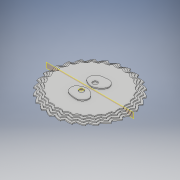
# Autodesk Inventor part: susuwatari
Saved by Autodesk Inventor 2018 (Build 220112000, 112)
## iProperties
Created: 2017-10-30
Part Number: susuwatari
Material: Generic
Document SubType Name: Modeling
Designer: lewisw19
Density: 1 g/cm^3
Appearance: Default
Author: lewisw19
Autodesk Inventor part; units mm, degrees
ref_plane "YZ Plane" through (0, 0, 0) normal (1, 0, 0) x (0, 1, 0)
ref_plane "XZ Plane" through (0, 0, 0) normal (0, 1, 0) x (-1, 0, 0)
sketch "Sketch1" plane through (0, 0, 0) normal (0, 1, 0) x (-1, 0, 0)
  arc A0 (255.3081, 0.1624) -> (269.4241, 48.2355) centre (181.7679, 47.8654) ccw
  arc A1 (248.6593, 60.0433) -> (269.4241, 48.2355) centre (269.4545, 72.4509) ccw
  arc A2 (248.6593, 60.0433) -> (250.9174, 108.9566) centre (165.7093, 88.3816) ccw
  arc A3 (228.0167, 115.6292) -> (250.9174, 108.9566) centre (245.3625, 132.5263) ccw
  arc A4 (228.0167, 115.6292) -> (218.9338, 163.7448) centre (140.7674, 124.074) ccw
  arc A5 (195.1456, 164.9347) -> (218.9338, 163.7448) centre (208.0931, 185.3981) ccw
  arc A6 (195.1456, 164.9347) -> (175.2114, 209.6586) centre (108.3007, 153.0308) ccw
  arc A7 (151.829, 205.3171) -> (175.2114, 209.6586) centre (159.6693, 228.2283) ccw
  arc A8 (151.829, 205.3171) -> (122.1181, 244.2383) centre (70.0702, 173.7063) ccw
  arc A9 (100.4094, 234.6175) -> (122.1181, 244.2383) centre (102.7124, 258.7232) ccw
  arc A10 (100.4094, 234.6175) -> (62.5234, 265.6378) centre (28.1443, 185.0038) ccw
  arc A11 (43.6616, 251.2759) -> (62.5234, 265.6378) centre (40.3004, 275.2569) ccw
  arc A12 (43.6616, 251.2759) -> (-0.3569, 272.7229) centre (-15.2139, 186.3341) ccw
  arc A13 (-15.3568, 254.4145) -> (-0.3569, 272.7229) centre (-24.1992, 276.9578) ccw
  arc A14 (-15.3568, 254.4145) -> (-63.1348, 265.132) centre (-57.6686, 177.6456) ccw
  arc A15 (-73.4706, 243.884) -> (-63.1348, 265.132) centre (-87.311, 263.7543) ccw
  arc A16 (-73.4706, 243.884) -> (-122.4324, 243.2943) centre (-96.9378, 159.4266) ccw
  arc A17 (-127.5582, 220.2704) -> (-122.4324, 243.2943) centre (-145.6392, 236.3783) ccw
  arc A18 (-127.5582, 220.2704) -> (-175.0642, 208.4052) centre (-130.9156, 132.6777) ccw
  arc A19 (-174.7194, 184.8623) -> (-175.0642, 208.4052) centre (-196.0506, 196.3238) ccw
  arc A20 (-174.7194, 184.8623) -> (-218.2085, 162.3613) centre (-157.786, 98.8564) ccw
  arc A21 (-212.4309, 139.5804) -> (-218.2085, 162.3613) centre (-235.8431, 145.7657) ccw
  arc A22 (-212.4309, 139.5804) -> (-249.5587, 107.6566) centre (-176.1197, 59.7979) ccw
  arc A23 (-238.6819, 86.8731) -> (-249.5587, 107.6566) centre (-262.8907, 87.4416) ccw
  arc A24 (-238.6819, 86.8731) -> (-267.4468, 47.2476) centre (-184.9504, 17.6151) ccw
  arc A25 (-252.0702, 29.5327) -> (-267.4468, 47.2476) centre (-275.7576, 24.5029) ccw
  arc A26 (-252.0702, 29.5327) -> (-267.6415, 0.1624) centre (-183.815, -25.4671) ccw
  arc A27 (269.4241, -47.9107) -> (255.3081, 0.1624) centre (181.7679, -47.5406) ccw
  arc A28 (269.4241, -47.9107) -> (248.6593, -59.7185) centre (269.4545, -72.1261) ccw
  arc A29 (250.9174, -108.6318) -> (248.6593, -59.7185) centre (165.7093, -88.0568) ccw
  arc A30 (250.9174, -108.6318) -> (228.0167, -115.3044) centre (245.3625, -132.2015) ccw
  arc A31 (218.9338, -163.42) -> (228.0167, -115.3044) centre (140.7674, -123.7492) ccw
  arc A32 (218.9338, -163.42) -> (195.1456, -164.6099) centre (208.0931, -185.0733) ccw
  arc A33 (175.2114, -209.3338) -> (195.1456, -164.6099) centre (108.3007, -152.706) ccw
  arc A34 (175.2114, -209.3338) -> (151.829, -204.9923) centre (159.6693, -227.9035) ccw
  arc A35 (122.1181, -243.9135) -> (151.829, -204.9923) centre (70.0702, -173.3815) ccw
  arc A36 (122.1181, -243.9135) -> (100.4094, -234.2927) centre (102.7124, -258.3984) ccw
  arc A37 (62.5234, -265.313) -> (100.4094, -234.2927) centre (28.1443, -184.679) ccw
  arc A38 (62.5234, -265.313) -> (43.6616, -250.9511) centre (40.3004, -274.9321) ccw
  arc A39 (-0.3569, -272.3981) -> (43.6616, -250.9511) centre (-15.2139, -186.0093) ccw
  arc A40 (-0.3569, -272.3981) -> (-15.3568, -254.0897) centre (-24.1992, -276.633) ccw
  arc A41 (-63.1348, -264.8072) -> (-15.3568, -254.0897) centre (-57.6686, -177.3208) ccw
  arc A42 (-63.1348, -264.8072) -> (-73.4706, -243.5592) centre (-87.311, -263.4295) ccw
  arc A43 (-122.4324, -242.9695) -> (-73.4706, -243.5592) centre (-96.9378, -159.1018) ccw
  arc A44 (-122.4324, -242.9695) -> (-127.5582, -219.9456) centre (-145.6392, -236.0535) ccw
  arc A45 (-175.0642, -208.0804) -> (-127.5582, -219.9456) centre (-130.9156, -132.3529) ccw
  arc A46 (-175.0642, -208.0804) -> (-174.7194, -184.5375) centre (-196.0506, -195.999) ccw
  arc A47 (-218.2085, -162.0365) -> (-174.7194, -184.5375) centre (-157.786, -98.5316) ccw
  arc A48 (-218.2085, -162.0365) -> (-212.4309, -139.2556) centre (-235.8431, -145.4409) ccw
  arc A49 (-249.5587, -107.3318) -> (-212.4309, -139.2556) centre (-176.1197, -59.4731) ccw
  arc A50 (-249.5587, -107.3318) -> (-238.6819, -86.5483) centre (-262.8907, -87.1168) ccw
  arc A51 (-267.4468, -46.9228) -> (-238.6819, -86.5483) centre (-184.9504, -17.2903) ccw
  arc A52 (-267.4468, -46.9228) -> (-252.0702, -29.2079) centre (-275.7576, -24.1781) ccw
  arc A53 (-267.6415, 0.1624) -> (-252.0702, -29.2079) centre (-183.815, 25.7919) ccw
  point P0 (0, 0)
  constraints: 108 point on circle, 54 centre point
extrude "Extrusion1" add sketch "Sketch1" along normal blind 6.35
sketch "Sketch2" plane through (0, 6.35, 0) normal (0, 1, 0) x (1, 0, 0)
  arc A0 (-255.3081, -0.1624) -> (-269.4241, -48.2355) centre (-181.7679, -47.8654) ccw projected
  arc A1 (-248.6593, -60.0433) -> (-269.4241, -48.2355) centre (-269.4545, -72.4509) ccw projected
  arc A2 (-248.6593, -60.0433) -> (-250.9174, -108.9566) centre (-165.7093, -88.3816) ccw projected
  arc A3 (-228.0167, -115.6292) -> (-250.9174, -108.9566) centre (-245.3625, -132.5263) ccw projected
  arc A4 (-228.0167, -115.6292) -> (-218.9338, -163.7448) centre (-140.7674, -124.074) ccw projected
  arc A5 (-195.1456, -164.9347) -> (-218.9338, -163.7448) centre (-208.0931, -185.3981) ccw projected
  arc A6 (-195.1456, -164.9347) -> (-175.2114, -209.6586) centre (-108.3007, -153.0308) ccw projected
  arc A7 (-151.829, -205.3171) -> (-175.2114, -209.6586) centre (-159.6693, -228.2283) ccw projected
  arc A8 (-151.829, -205.3171) -> (-122.1181, -244.2383) centre (-70.0702, -173.7063) ccw projected
  arc A9 (-100.4094, -234.6175) -> (-122.1181, -244.2383) centre (-102.7124, -258.7232) ccw projected
  arc A10 (-100.4094, -234.6175) -> (-62.5234, -265.6378) centre (-28.1443, -185.0038) ccw projected
  arc A11 (-43.6616, -251.2759) -> (-62.5234, -265.6378) centre (-40.3004, -275.2569) ccw projected
  arc A12 (-43.6616, -251.2759) -> (0.3569, -272.7229) centre (15.2139, -186.3341) ccw projected
  arc A13 (15.3568, -254.4145) -> (0.3569, -272.7229) centre (24.1992, -276.9578) ccw projected
  arc A14 (15.3568, -254.4145) -> (63.1348, -265.132) centre (57.6686, -177.6456) ccw projected
  arc A15 (73.4706, -243.884) -> (63.1348, -265.132) centre (87.311, -263.7543) ccw projected
  arc A16 (73.4706, -243.884) -> (122.4324, -243.2943) centre (96.9378, -159.4266) ccw projected
  arc A17 (127.5582, -220.2704) -> (122.4324, -243.2943) centre (145.6392, -236.3783) ccw projected
  arc A18 (127.5582, -220.2704) -> (175.0642, -208.4052) centre (130.9156, -132.6777) ccw projected
  arc A19 (174.7194, -184.8623) -> (175.0642, -208.4052) centre (196.0506, -196.3238) ccw projected
  arc A20 (174.7194, -184.8623) -> (218.2085, -162.3613) centre (157.786, -98.8564) ccw projected
  arc A21 (212.4309, -139.5804) -> (218.2085, -162.3613) centre (235.8431, -145.7657) ccw projected
  arc A22 (212.4309, -139.5804) -> (249.5587, -107.6566) centre (176.1197, -59.7979) ccw projected
  arc A23 (238.6819, -86.8731) -> (249.5587, -107.6566) centre (262.8907, -87.4416) ccw projected
  arc A24 (238.6819, -86.8731) -> (267.4468, -47.2476) centre (184.9504, -17.6151) ccw projected
  arc A25 (252.0702, -29.5327) -> (267.4468, -47.2476) centre (275.7576, -24.5029) ccw projected
  arc A26 (252.0702, -29.5327) -> (267.6415, -0.1624) centre (183.815, 25.4671) ccw projected
  arc A27 (267.6415, -0.1624) -> (252.0702, 29.2079) centre (183.815, -25.7919) ccw projected
  arc A28 (267.4468, 46.9228) -> (252.0702, 29.2079) centre (275.7576, 24.1781) ccw projected
  arc A29 (267.4468, 46.9228) -> (238.6819, 86.5483) centre (184.9504, 17.2903) ccw projected
  arc A30 (249.5587, 107.3318) -> (238.6819, 86.5483) centre (262.8907, 87.1168) ccw projected
  arc A31 (249.5587, 107.3318) -> (212.4309, 139.2556) centre (176.1197, 59.4731) ccw projected
  arc A32 (218.2085, 162.0365) -> (212.4309, 139.2556) centre (235.8431, 145.4409) ccw projected
  arc A33 (218.2085, 162.0365) -> (174.7194, 184.5375) centre (157.786, 98.5316) ccw projected
  arc A34 (175.0642, 208.0804) -> (174.7194, 184.5375) centre (196.0506, 195.999) ccw projected
  arc A35 (175.0642, 208.0804) -> (127.5582, 219.9456) centre (130.9156, 132.3529) ccw projected
  arc A36 (122.4324, 242.9695) -> (127.5582, 219.9456) centre (145.6392, 236.0535) ccw projected
  arc A37 (122.4324, 242.9695) -> (73.4706, 243.5592) centre (96.9378, 159.1018) ccw projected
  arc A38 (63.1348, 264.8072) -> (73.4706, 243.5592) centre (87.311, 263.4295) ccw projected
  arc A39 (63.1348, 264.8072) -> (15.3568, 254.0897) centre (57.6686, 177.3208) ccw projected
  arc A40 (0.3569, 272.3981) -> (15.3568, 254.0897) centre (24.1992, 276.633) ccw projected
  arc A41 (0.3569, 272.3981) -> (-43.6616, 250.9511) centre (15.2139, 186.0093) ccw projected
  arc A42 (-62.5234, 265.313) -> (-43.6616, 250.9511) centre (-40.3004, 274.9321) ccw projected
  arc A43 (-62.5234, 265.313) -> (-100.4094, 234.2927) centre (-28.1443, 184.679) ccw projected
  arc A44 (-122.1181, 243.9135) -> (-100.4094, 234.2927) centre (-102.7124, 258.3984) ccw projected
  arc A45 (-122.1181, 243.9135) -> (-151.829, 204.9923) centre (-70.0702, 173.3815) ccw projected
  arc A46 (-175.2114, 209.3338) -> (-151.829, 204.9923) centre (-159.6693, 227.9035) ccw projected
  arc A47 (-175.2114, 209.3338) -> (-195.1456, 164.6099) centre (-108.3007, 152.706) ccw projected
  arc A48 (-218.9338, 163.42) -> (-195.1456, 164.6099) centre (-208.0931, 185.0733) ccw projected
  arc A49 (-218.9338, 163.42) -> (-228.0167, 115.3044) centre (-140.7674, 123.7492) ccw projected
  arc A50 (-250.9174, 108.6318) -> (-228.0167, 115.3044) centre (-245.3625, 132.2015) ccw projected
  arc A51 (-250.9174, 108.6318) -> (-248.6593, 59.7185) centre (-165.7093, 88.0568) ccw projected
  arc A52 (-269.4241, 47.9107) -> (-248.6593, 59.7185) centre (-269.4545, 72.1261) ccw projected
  arc A53 (-269.4241, 47.9107) -> (-255.3081, -0.1624) centre (-181.7679, 47.5406) ccw projected
  arc A54 (-234.8822, -59.5084) -> (-240.282, -95.9621) centre (-165.7093, -88.3816) ccw
  arc A55 (-234.8822, -59.5084) -> (-256.0786, -38.044) centre (-269.4545, -72.4509) ccw
  arc A56 (-239.5863, -0.1624) -> (-256.0786, -38.044) centre (-181.7679, -47.8654) ccw
  arc A57 (-256.0786, 37.7192) -> (-239.5863, -0.1624) centre (-181.7679, 47.5406) ccw
  arc A58 (-256.0786, 37.7192) -> (-234.8822, 59.1836) centre (-269.4545, 72.1261) ccw
  arc A59 (-240.282, 95.6373) -> (-234.8822, 59.1836) centre (-165.7093, 88.0568) ccw
  arc A60 (-240.282, 95.6373) -> (-214.7327, 111.5965) centre (-245.3625, 132.2015) ccw
  arc A61 (-211.5818, 148.3231) -> (-214.7327, 111.5965) centre (-140.7674, 123.7492) ccw
  arc A62 (-211.5818, 148.3231) -> (-183.0755, 157.9279) centre (-208.0931, 185.0733) ccw
  arc A63 (-171.5391, 192.9484) -> (-183.0755, 157.9279) centre (-108.3007, 152.706) ccw
  arc A64 (-171.5391, 192.9484) -> (-141.6285, 195.6966) centre (-159.6693, 227.9035) ccw
  arc A65 (-122.3236, 227.1229) -> (-141.6285, 195.6966) centre (-70.0702, 173.3815) ccw
  arc A66 (-122.3236, 227.1229) -> (-92.6332, 222.8856) centre (-102.7124, 258.3984) ccw
  arc A67 (-66.5955, 249.0223) -> (-92.6332, 222.8856) centre (-28.1443, 184.679) ccw
  arc A68 (-66.5955, 249.0223) -> (-38.7336, 238.0499) centre (-40.3004, 274.9321) ccw
  arc A69 (-7.3623, 257.4856) -> (-38.7336, 238.0499) centre (15.2139, 186.0093) ccw
  arc A70 (-7.3623, 257.4856) -> (17.1669, 240.3935) centre (24.1992, 276.633) ccw
  arc A71 (52.1846, 252.0769) -> (17.1669, 240.3935) centre (57.6686, 177.3208) ccw
  arc A72 (52.1846, 252.0769) -> (72.0621, 229.8108) centre (87.311, 263.4295) ccw
  arc A73 (108.8415, 233.1076) -> (72.0621, 229.8108) centre (96.9378, 159.1018) ccw
  arc A74 (108.8415, 233.1076) -> (123.0048, 206.8913) centre (145.6392, 236.0535) ccw
  arc A75 (159.5654, 201.6187) -> (123.0048, 206.8913) centre (130.9156, 132.3529) ccw
  arc A76 (159.5654, 201.6187) -> (167.2656, 172.8868) centre (196.0506, 195.999) ccw
  arc A77 (201.6373, 159.3232) -> (167.2656, 172.8868) centre (157.786, 98.5316) ccw
  arc A78 (201.6373, 159.3232) -> (202.479, 129.6424) centre (235.8431, 145.4409) ccw
  arc A79 (232.8084, 108.5132) -> (202.479, 129.6424) centre (176.1197, 59.4731) ccw
  arc A80 (232.8084, 108.5132) -> (226.7703, 79.4968) centre (262.8907, 87.1168) ccw
  arc A81 (251.4205, 51.9353) -> (226.7703, 79.4968) centre (184.9504, 17.2903) ccw
  arc A82 (251.4205, 51.9353) -> (238.8535, 25.0935) centre (275.7576, 24.1781) ccw
  arc A83 (254.2542, -0.1624) -> (238.8535, 25.0935) centre (183.815, -25.7919) ccw
  arc A84 (238.8535, -25.4183) -> (254.2542, -0.1624) centre (183.815, 25.4671) ccw
  arc A85 (238.8535, -25.4183) -> (251.4205, -52.2601) centre (275.7576, -24.5029) ccw
  arc A86 (226.7703, -79.8216) -> (251.4205, -52.2601) centre (184.9504, -17.6151) ccw
  arc A87 (226.7703, -79.8216) -> (232.8084, -108.838) centre (262.8907, -87.4416) ccw
  arc A88 (202.479, -129.9672) -> (232.8084, -108.838) centre (176.1197, -59.7979) ccw
  arc A89 (202.479, -129.9672) -> (201.6373, -159.648) centre (235.8431, -145.7657) ccw
  arc A90 (167.2656, -173.2116) -> (201.6373, -159.648) centre (157.786, -98.8564) ccw
  arc A91 (167.2656, -173.2116) -> (159.5654, -201.9435) centre (196.0506, -196.3238) ccw
  arc A92 (123.0048, -207.2161) -> (159.5654, -201.9435) centre (130.9156, -132.6777) ccw
  arc A93 (123.0048, -207.2161) -> (108.8415, -233.4324) centre (145.6392, -236.3783) ccw
  arc A94 (72.0621, -230.1356) -> (108.8415, -233.4324) centre (96.9378, -159.4266) ccw
  arc A95 (72.0621, -230.1356) -> (52.1846, -252.4017) centre (87.311, -263.7543) ccw
  arc A96 (17.1669, -240.7183) -> (52.1846, -252.4017) centre (57.6686, -177.6456) ccw
  arc A97 (17.1669, -240.7183) -> (-7.3623, -257.8104) centre (24.1992, -276.9578) ccw
  arc A98 (-38.7336, -238.3747) -> (-7.3623, -257.8104) centre (15.2139, -186.3341) ccw
  arc A99 (-38.7336, -238.3747) -> (-66.5955, -249.3471) centre (-40.3004, -275.2569) ccw
  arc A100 (-92.6332, -223.2104) -> (-66.5955, -249.3471) centre (-28.1443, -185.0038) ccw
  arc A101 (-92.6332, -223.2104) -> (-122.3236, -227.4477) centre (-102.7124, -258.7232) ccw
  arc A102 (-141.6285, -196.0214) -> (-122.3236, -227.4477) centre (-70.0702, -173.7063) ccw
  arc A103 (-141.6285, -196.0214) -> (-171.5391, -193.2732) centre (-159.6693, -228.2283) ccw
  arc A104 (-183.0755, -158.2527) -> (-171.5391, -193.2732) centre (-108.3007, -153.0308) ccw
  arc A105 (-183.0755, -158.2527) -> (-211.5818, -148.6479) centre (-208.0931, -185.3981) ccw
  arc A106 (-214.7327, -111.9213) -> (-211.5818, -148.6479) centre (-140.7674, -124.074) ccw
  arc A107 (-214.7327, -111.9213) -> (-240.282, -95.9621) centre (-245.3625, -132.5263) ccw
  point P0 (0, 0)
  dimension "d10" = 12.7
  constraints: 108 point on circle, 54 centre point, 53 other
  measures "d10" radial gap between concentric circles of A3 A107
extrude "Extrusion2" add sketch "Sketch2" along normal blind 6.35 contours A55 A56 A57 A58 A59 A60 A61 A62 A63 A64 A65 A66 A67 A68 A69 A70 A71 A72 A73 A74 A75 A76 A77 A78 A79 A80 A81 A82 A83 A84 A85 A86 A87 A88 A89 A90 A91 A92 A93 A94 A95 A96 A97 A98 A99 A100 A101 A102 A103 A104 A105 A106 A107 A54
sketch "Sketch3" plane through (0, 12.7, 0) normal (0, 1, 0) x (1, 0, 0)
  arc A0 (-234.8822, -59.5084) -> (-240.282, -95.9621) centre (-165.7093, -88.3816) ccw projected
  arc A1 (-214.7327, -111.9213) -> (-240.282, -95.9621) centre (-245.3625, -132.5263) ccw projected
  arc A2 (-214.7327, -111.9213) -> (-211.5818, -148.6479) centre (-140.7674, -124.074) ccw projected
  arc A3 (-183.0755, -158.2527) -> (-211.5818, -148.6479) centre (-208.0931, -185.3981) ccw projected
  arc A4 (-183.0755, -158.2527) -> (-171.5391, -193.2732) centre (-108.3007, -153.0308) ccw projected
  arc A5 (-141.6285, -196.0214) -> (-171.5391, -193.2732) centre (-159.6693, -228.2283) ccw projected
  arc A6 (-141.6285, -196.0214) -> (-122.3236, -227.4477) centre (-70.0702, -173.7063) ccw projected
  arc A7 (-92.6332, -223.2104) -> (-122.3236, -227.4477) centre (-102.7124, -258.7232) ccw projected
  arc A8 (-92.6332, -223.2104) -> (-66.5955, -249.3471) centre (-28.1443, -185.0038) ccw projected
  arc A9 (-38.7336, -238.3747) -> (-66.5955, -249.3471) centre (-40.3004, -275.2569) ccw projected
  arc A10 (-38.7336, -238.3747) -> (-7.3623, -257.8104) centre (15.2139, -186.3341) ccw projected
  arc A11 (17.1669, -240.7183) -> (-7.3623, -257.8104) centre (24.1992, -276.9578) ccw projected
  arc A12 (17.1669, -240.7183) -> (52.1846, -252.4017) centre (57.6686, -177.6456) ccw projected
  arc A13 (72.0621, -230.1356) -> (52.1846, -252.4017) centre (87.311, -263.7543) ccw projected
  arc A14 (72.0621, -230.1356) -> (108.8415, -233.4324) centre (96.9378, -159.4266) ccw projected
  arc A15 (123.0048, -207.2161) -> (108.8415, -233.4324) centre (145.6392, -236.3783) ccw projected
  arc A16 (123.0048, -207.2161) -> (159.5654, -201.9435) centre (130.9156, -132.6777) ccw projected
  arc A17 (167.2656, -173.2116) -> (159.5654, -201.9435) centre (196.0506, -196.3238) ccw projected
  arc A18 (167.2656, -173.2116) -> (201.6373, -159.648) centre (157.786, -98.8564) ccw projected
  arc A19 (202.479, -129.9672) -> (201.6373, -159.648) centre (235.8431, -145.7657) ccw projected
  arc A20 (202.479, -129.9672) -> (232.8084, -108.838) centre (176.1197, -59.7979) ccw projected
  arc A21 (226.7703, -79.8216) -> (232.8084, -108.838) centre (262.8907, -87.4416) ccw projected
  arc A22 (226.7703, -79.8216) -> (251.4205, -52.2601) centre (184.9504, -17.6151) ccw projected
  arc A23 (238.8535, -25.4183) -> (251.4205, -52.2601) centre (275.7576, -24.5029) ccw projected
  arc A24 (238.8535, -25.4183) -> (254.2542, -0.1624) centre (183.815, 25.4671) ccw projected
  arc A25 (254.2542, -0.1624) -> (238.8535, 25.0935) centre (183.815, -25.7919) ccw projected
  arc A26 (251.4205, 51.9353) -> (238.8535, 25.0935) centre (275.7576, 24.1781) ccw projected
  arc A27 (251.4205, 51.9353) -> (226.7703, 79.4968) centre (184.9504, 17.2903) ccw projected
  arc A28 (232.8084, 108.5132) -> (226.7703, 79.4968) centre (262.8907, 87.1168) ccw projected
  arc A29 (232.8084, 108.5132) -> (202.479, 129.6424) centre (176.1197, 59.4731) ccw projected
  arc A30 (201.6373, 159.3232) -> (202.479, 129.6424) centre (235.8431, 145.4409) ccw projected
  arc A31 (201.6373, 159.3232) -> (167.2656, 172.8868) centre (157.786, 98.5316) ccw projected
  arc A32 (159.5654, 201.6187) -> (167.2656, 172.8868) centre (196.0506, 195.999) ccw projected
  arc A33 (159.5654, 201.6187) -> (123.0048, 206.8913) centre (130.9156, 132.3529) ccw projected
  arc A34 (108.8415, 233.1076) -> (123.0048, 206.8913) centre (145.6392, 236.0535) ccw projected
  arc A35 (108.8415, 233.1076) -> (72.0621, 229.8108) centre (96.9378, 159.1018) ccw projected
  arc A36 (52.1846, 252.0769) -> (72.0621, 229.8108) centre (87.311, 263.4295) ccw projected
  arc A37 (52.1846, 252.0769) -> (17.1669, 240.3935) centre (57.6686, 177.3208) ccw projected
  arc A38 (-7.3623, 257.4856) -> (17.1669, 240.3935) centre (24.1992, 276.633) ccw projected
  arc A39 (-7.3623, 257.4856) -> (-38.7336, 238.0499) centre (15.2139, 186.0093) ccw projected
  arc A40 (-66.5955, 249.0223) -> (-38.7336, 238.0499) centre (-40.3004, 274.9321) ccw projected
  arc A41 (-66.5955, 249.0223) -> (-92.6332, 222.8856) centre (-28.1443, 184.679) ccw projected
  arc A42 (-122.3236, 227.1229) -> (-92.6332, 222.8856) centre (-102.7124, 258.3984) ccw projected
  arc A43 (-122.3236, 227.1229) -> (-141.6285, 195.6966) centre (-70.0702, 173.3815) ccw projected
  arc A44 (-171.5391, 192.9484) -> (-141.6285, 195.6966) centre (-159.6693, 227.9035) ccw projected
  arc A45 (-171.5391, 192.9484) -> (-183.0755, 157.9279) centre (-108.3007, 152.706) ccw projected
  arc A46 (-211.5818, 148.3231) -> (-183.0755, 157.9279) centre (-208.0931, 185.0733) ccw projected
  arc A47 (-211.5818, 148.3231) -> (-214.7327, 111.5965) centre (-140.7674, 123.7492) ccw projected
  arc A48 (-240.282, 95.6373) -> (-214.7327, 111.5965) centre (-245.3625, 132.2015) ccw projected
  arc A49 (-240.282, 95.6373) -> (-234.8822, 59.1836) centre (-165.7093, 88.0568) ccw projected
  arc A50 (-256.0786, 37.7192) -> (-234.8822, 59.1836) centre (-269.4545, 72.1261) ccw projected
  arc A51 (-256.0786, 37.7192) -> (-239.5863, -0.1624) centre (-181.7679, 47.5406) ccw projected
  arc A52 (-239.5863, -0.1624) -> (-256.0786, -38.044) centre (-181.7679, -47.8654) ccw projected
  arc A53 (-234.8822, -59.5084) -> (-256.0786, -38.044) centre (-269.4545, -72.4509) ccw projected
  arc A54 (-119.2108, 211.6063) -> (-130.6715, 187.644) centre (-70.0702, 173.3815) ccw
  arc A55 (-119.2108, 211.6063) -> (-83.8313, 212.516) centre (-102.7124, 258.3984) ccw
  arc A56 (-67.1451, 233.2061) -> (-83.8313, 212.516) centre (-28.1443, 184.679) ccw
  arc A57 (-67.1451, 233.2061) -> (-32.5648, 225.9234) centre (-40.3004, 274.9321) ccw
  arc A58 (-11.5445, 242.2225) -> (-32.5648, 225.9234) centre (15.2139, 186.0093) ccw
  arc A59 (-11.5445, 242.2225) -> (20.3669, 227.1657) centre (24.1992, 276.633) ccw
  arc A60 (44.5952, 238.1897) -> (20.3669, 227.1657) centre (57.6686, 177.3208) ccw
  arc A61 (44.5952, 238.1897) -> (72.118, 216.1975) centre (87.311, 263.4295) ccw
  arc A62 (98.2541, 221.3449) -> (72.118, 216.1975) centre (96.9378, 159.1018) ccw
  arc A63 (98.2541, 221.3449) -> (119.9116, 193.6297) centre (145.6392, 236.0535) ccw
  arc A64 (146.5507, 192.6147) -> (119.9116, 193.6297) centre (130.9156, 132.3529) ccw
  arc A65 (146.5507, 192.6147) -> (161.1886, 160.6955) centre (196.0506, 195.999) ccw
  arc A66 (186.897, 153.5633) -> (161.1886, 160.6955) centre (157.786, 98.5316) ccw
  arc A67 (186.897, 153.5633) -> (193.7454, 119.183) centre (235.8431, 145.4409) ccw
  arc A68 (217.1371, 106.308) -> (193.7454, 119.183) centre (176.1197, 59.4731) ccw
  arc A69 (217.1371, 106.308) -> (215.8514, 71.3372) centre (262.8907, 87.1168) ccw
  arc A70 (235.663, 53.4035) -> (215.8514, 71.3372) centre (184.9504, 17.2903) ccw
  arc A71 (235.663, 53.4035) -> (226.3472, 19.6718) centre (275.7576, 24.1781) ccw
  arc A72 (240.5518, -0.1624) -> (226.3472, 19.6718) centre (183.815, -25.7919) ccw
  arc A73 (226.3472, -19.9966) -> (240.5518, -0.1624) centre (183.815, 25.4671) ccw
  arc A74 (226.3472, -19.9966) -> (235.663, -53.7283) centre (275.7576, -24.5029) ccw
  arc A75 (215.8514, -71.662) -> (235.663, -53.7283) centre (184.9504, -17.6151) ccw
  arc A76 (215.8514, -71.662) -> (217.1371, -106.6328) centre (262.8907, -87.4416) ccw
  arc A77 (193.7454, -119.5077) -> (217.1371, -106.6328) centre (176.1197, -59.7979) ccw
  arc A78 (193.7454, -119.5077) -> (186.897, -153.8881) centre (235.8431, -145.7657) ccw
  arc A79 (161.1886, -161.0203) -> (186.897, -153.8881) centre (157.786, -98.8564) ccw
  arc A80 (161.1886, -161.0203) -> (146.5507, -192.9395) centre (196.0506, -196.3238) ccw
  arc A81 (119.9116, -193.9545) -> (146.5507, -192.9395) centre (130.9156, -132.6777) ccw
  arc A82 (119.9116, -193.9545) -> (98.2541, -221.6697) centre (145.6392, -236.3783) ccw
  arc A83 (72.118, -216.5223) -> (98.2541, -221.6697) centre (96.9378, -159.4266) ccw
  arc A84 (72.118, -216.5223) -> (44.5952, -238.5145) centre (87.311, -263.7543) ccw
  arc A85 (20.3669, -227.4905) -> (44.5952, -238.5145) centre (57.6686, -177.6456) ccw
  arc A86 (20.3669, -227.4905) -> (-11.5445, -242.5473) centre (24.1992, -276.9578) ccw
  arc A87 (-32.5648, -226.2482) -> (-11.5445, -242.5473) centre (15.2139, -186.3341) ccw
  arc A88 (-32.5648, -226.2482) -> (-67.1451, -233.5309) centre (-40.3004, -275.2569) ccw
  arc A89 (-83.8313, -212.8408) -> (-67.1451, -233.5309) centre (-28.1443, -185.0038) ccw
  arc A90 (-83.8313, -212.8408) -> (-119.2108, -211.9311) centre (-102.7124, -258.7232) ccw
  arc A91 (-130.6715, -187.9688) -> (-119.2108, -211.9311) centre (-70.0702, -173.7063) ccw
  arc A92 (-130.6715, -187.9688) -> (-164.9319, -178.8927) centre (-159.6693, -228.2283) ccw
  arc A93 (-170.5576, -152.9515) -> (-164.9319, -178.8927) centre (-108.3007, -153.0308) ccw
  arc A94 (-170.5576, -152.9515) -> (-201.8363, -136.1787) centre (-208.0931, -185.3981) ccw
  arc A95 (-201.3321, -109.6568) -> (-201.8363, -136.1787) centre (-140.7674, -124.074) ccw
  arc A96 (-201.3321, -109.6568) -> (-227.9236, -86.0765) centre (-245.3625, -132.5263) ccw
  arc A97 (-221.3244, -60.4013) -> (-227.9236, -86.0765) centre (-165.7093, -88.3816) ccw
  arc A98 (-221.3244, -60.4013) -> (-241.7736, -31.2749) centre (-269.4545, -72.4509) ccw
  arc A99 (-221.7723, -0.1624) -> (-241.7736, -31.2749) centre (-181.7679, -47.8654) ccw
  arc A100 (-241.7736, 30.9501) -> (-221.7723, -0.1624) centre (-181.7679, 47.5406) ccw
  arc A101 (-241.7736, 30.9501) -> (-221.3244, 60.0765) centre (-269.4545, 72.1261) ccw
  arc A102 (-227.9236, 85.7517) -> (-221.3244, 60.0765) centre (-165.7093, 88.0568) ccw
  arc A103 (-227.9236, 85.7517) -> (-201.3321, 109.332) centre (-245.3625, 132.2015) ccw
  arc A104 (-201.8363, 135.8539) -> (-201.3321, 109.332) centre (-140.7674, 123.7492) ccw
  arc A105 (-201.8363, 135.8539) -> (-170.5576, 152.6267) centre (-208.0931, 185.0733) ccw
  arc A106 (-164.9319, 178.5679) -> (-170.5576, 152.6267) centre (-108.3007, 152.706) ccw
  arc A107 (-164.9319, 178.5679) -> (-130.6715, 187.644) centre (-159.6693, 227.9035) ccw
  point P0 (0, 0)
  dimension "d13" = 12.7
  constraints: 108 point on circle, 54 centre point, 53 other
  measures "d13" radial gap between concentric circles of A44 A107
extrude "Extrusion3" add sketch "Sketch3" along normal blind 6.35 contours A55 A56 A57 A58 A59 A60 A61 A62 A63 A64 A65 A66 A67 A68 A69 A70 A71 A72 A73 A74 A75 A76 A77 A78 A79 A80 A81 A82 A83 A84 A85 A86 A87 A88 A89 A90 A91 A92 A93 A94 A95 A96 A97 A98 A99 A100 A101 A102 A103 A104 A105 A106 A107 A54
sketch "Sketch4" plane through (0, 19.05, 0) normal (0, 1, 0) x (1, 0, 0)
  arc A0 (-119.2108, 211.6063) -> (-130.6715, 187.644) centre (-70.0702, 173.3815) ccw projected
  arc A1 (-164.9319, 178.5679) -> (-130.6715, 187.644) centre (-159.6693, 227.9035) ccw projected
  arc A2 (-164.9319, 178.5679) -> (-170.5576, 152.6267) centre (-108.3007, 152.706) ccw projected
  arc A3 (-201.8363, 135.8539) -> (-170.5576, 152.6267) centre (-208.0931, 185.0733) ccw projected
  arc A4 (-201.8363, 135.8539) -> (-201.3321, 109.332) centre (-140.7674, 123.7492) ccw projected
  arc A5 (-227.9236, 85.7517) -> (-201.3321, 109.332) centre (-245.3625, 132.2015) ccw projected
  arc A6 (-227.9236, 85.7517) -> (-221.3244, 60.0765) centre (-165.7093, 88.0568) ccw projected
  arc A7 (-241.7736, 30.9501) -> (-221.3244, 60.0765) centre (-269.4545, 72.1261) ccw projected
  arc A8 (-241.7736, 30.9501) -> (-221.7723, -0.1624) centre (-181.7679, 47.5406) ccw projected
  arc A9 (-221.7723, -0.1624) -> (-241.7736, -31.2749) centre (-181.7679, -47.8654) ccw projected
  arc A10 (-221.3244, -60.4013) -> (-241.7736, -31.2749) centre (-269.4545, -72.4509) ccw projected
  arc A11 (-221.3244, -60.4013) -> (-227.9236, -86.0765) centre (-165.7093, -88.3816) ccw projected
  arc A12 (-201.3321, -109.6568) -> (-227.9236, -86.0765) centre (-245.3625, -132.5263) ccw projected
  arc A13 (-201.3321, -109.6568) -> (-201.8363, -136.1787) centre (-140.7674, -124.074) ccw projected
  arc A14 (-170.5576, -152.9515) -> (-201.8363, -136.1787) centre (-208.0931, -185.3981) ccw projected
  arc A15 (-170.5576, -152.9515) -> (-164.9319, -178.8927) centre (-108.3007, -153.0308) ccw projected
  arc A16 (-130.6715, -187.9688) -> (-164.9319, -178.8927) centre (-159.6693, -228.2283) ccw projected
  arc A17 (-130.6715, -187.9688) -> (-119.2108, -211.9311) centre (-70.0702, -173.7063) ccw projected
  arc A18 (-83.8313, -212.8408) -> (-119.2108, -211.9311) centre (-102.7124, -258.7232) ccw projected
  arc A19 (-83.8313, -212.8408) -> (-67.1451, -233.5309) centre (-28.1443, -185.0038) ccw projected
  arc A20 (-32.5648, -226.2482) -> (-67.1451, -233.5309) centre (-40.3004, -275.2569) ccw projected
  arc A21 (-32.5648, -226.2482) -> (-11.5445, -242.5473) centre (15.2139, -186.3341) ccw projected
  arc A22 (20.3669, -227.4905) -> (-11.5445, -242.5473) centre (24.1992, -276.9578) ccw projected
  arc A23 (20.3669, -227.4905) -> (44.5952, -238.5145) centre (57.6686, -177.6456) ccw projected
  arc A24 (72.118, -216.5223) -> (44.5952, -238.5145) centre (87.311, -263.7543) ccw projected
  arc A25 (72.118, -216.5223) -> (98.2541, -221.6697) centre (96.9378, -159.4266) ccw projected
  arc A26 (119.9116, -193.9545) -> (98.2541, -221.6697) centre (145.6392, -236.3783) ccw projected
  arc A27 (119.9116, -193.9545) -> (146.5507, -192.9395) centre (130.9156, -132.6777) ccw projected
  arc A28 (161.1886, -161.0203) -> (146.5507, -192.9395) centre (196.0506, -196.3238) ccw projected
  arc A29 (161.1886, -161.0203) -> (186.897, -153.8881) centre (157.786, -98.8564) ccw projected
  arc A30 (193.7454, -119.5077) -> (186.897, -153.8881) centre (235.8431, -145.7657) ccw projected
  arc A31 (193.7454, -119.5077) -> (217.1371, -106.6328) centre (176.1197, -59.7979) ccw projected
  arc A32 (215.8514, -71.662) -> (217.1371, -106.6328) centre (262.8907, -87.4416) ccw projected
  arc A33 (215.8514, -71.662) -> (235.663, -53.7283) centre (184.9504, -17.6151) ccw projected
  arc A34 (226.3472, -19.9966) -> (235.663, -53.7283) centre (275.7576, -24.5029) ccw projected
  arc A35 (226.3472, -19.9966) -> (240.5518, -0.1624) centre (183.815, 25.4671) ccw projected
  arc A36 (240.5518, -0.1624) -> (226.3472, 19.6718) centre (183.815, -25.7919) ccw projected
  arc A37 (235.663, 53.4035) -> (226.3472, 19.6718) centre (275.7576, 24.1781) ccw projected
  arc A38 (235.663, 53.4035) -> (215.8514, 71.3372) centre (184.9504, 17.2903) ccw projected
  arc A39 (217.1371, 106.308) -> (215.8514, 71.3372) centre (262.8907, 87.1168) ccw projected
  arc A40 (217.1371, 106.308) -> (193.7454, 119.183) centre (176.1197, 59.4731) ccw projected
  arc A41 (186.897, 153.5633) -> (193.7454, 119.183) centre (235.8431, 145.4409) ccw projected
  arc A42 (186.897, 153.5633) -> (161.1886, 160.6955) centre (157.786, 98.5316) ccw projected
  arc A43 (146.5507, 192.6147) -> (161.1886, 160.6955) centre (196.0506, 195.999) ccw projected
  arc A44 (146.5507, 192.6147) -> (119.9116, 193.6297) centre (130.9156, 132.3529) ccw projected
  arc A45 (98.2541, 221.3449) -> (119.9116, 193.6297) centre (145.6392, 236.0535) ccw projected
  arc A46 (98.2541, 221.3449) -> (72.118, 216.1975) centre (96.9378, 159.1018) ccw projected
  arc A47 (44.5952, 238.1897) -> (72.118, 216.1975) centre (87.311, 263.4295) ccw projected
  arc A48 (44.5952, 238.1897) -> (20.3669, 227.1657) centre (57.6686, 177.3208) ccw projected
  arc A49 (-11.5445, 242.2225) -> (20.3669, 227.1657) centre (24.1992, 276.633) ccw projected
  arc A50 (-11.5445, 242.2225) -> (-32.5648, 225.9234) centre (15.2139, 186.0093) ccw projected
  arc A51 (-67.1451, 233.2061) -> (-32.5648, 225.9234) centre (-40.3004, 274.9321) ccw projected
  arc A52 (-67.1451, 233.2061) -> (-83.8313, 212.516) centre (-28.1443, 184.679) ccw projected
  arc A53 (-119.2108, 211.6063) -> (-83.8313, 212.516) centre (-102.7124, 258.3984) ccw projected
  arc A54 (-65.0567, 217.7452) -> (-74.1937, 202.9917) centre (-28.1443, 184.679) ccw
  arc A55 (-65.0567, 217.7452) -> (-25.3851, 214.428) centre (-40.3004, 274.9321) ccw
  arc A56 (-13.078, 226.6967) -> (-25.3851, 214.428) centre (15.2139, 186.0093) ccw
  arc A57 (-13.078, 226.6967) -> (24.6991, 214.3195) centre (24.1992, 276.633) ccw
  arc A58 (39.5226, 223.4361) -> (24.6991, 214.3195) centre (57.6686, 177.3208) ccw
  arc A59 (39.5226, 223.4361) -> (73.3667, 202.6943) centre (87.311, 263.4295) ccw
  arc A60 (89.9158, 208.1588) -> (73.3667, 202.6943) centre (96.9378, 159.1018) ccw
  arc A61 (89.9158, 208.1588) -> (118.0074, 180.1993) centre (145.6392, 236.0535) ccw
  arc A62 (135.3962, 181.7069) -> (118.0074, 180.1993) centre (130.9156, 132.3529) ccw
  arc A63 (135.3962, 181.7069) -> (156.2326, 148.0642) centre (196.0506, 195.999) ccw
  arc A64 (173.5277, 145.522) -> (156.2326, 148.0642) centre (157.786, 98.5316) ccw
  arc A65 (173.5277, 145.522) -> (186.0036, 108.0344) centre (235.8431, 145.4409) ccw
  arc A66 (202.2737, 101.5666) -> (186.0036, 108.0344) centre (176.1197, 59.4731) ccw
  arc A67 (202.2737, 101.5666) -> (205.7407, 62.2754) centre (262.8907, 87.1168) ccw
  arc A68 (220.1069, 52.2176) -> (205.7407, 62.2754) centre (184.9504, 17.2903) ccw
  arc A69 (220.1069, 52.2176) -> (214.4192, 13.186) centre (275.7576, 24.1781) ccw
  arc A70 (226.2299, -0.1624) -> (214.4192, 13.186) centre (183.815, -25.7919) ccw
  arc A71 (214.4192, -13.5108) -> (226.2299, -0.1624) centre (183.815, 25.4671) ccw
  arc A72 (214.4192, -13.5108) -> (220.1069, -52.5424) centre (275.7576, -24.5029) ccw
  arc A73 (205.7407, -62.6002) -> (220.1069, -52.5424) centre (184.9504, -17.6151) ccw
  arc A74 (205.7407, -62.6002) -> (202.2737, -101.8914) centre (262.8907, -87.4416) ccw
  arc A75 (186.0036, -108.3592) -> (202.2737, -101.8914) centre (176.1197, -59.7979) ccw
  arc A76 (186.0036, -108.3592) -> (173.5277, -145.8468) centre (235.8431, -145.7657) ccw
  arc A77 (156.2326, -148.389) -> (173.5277, -145.8468) centre (157.786, -98.8564) ccw
  arc A78 (156.2326, -148.389) -> (135.3962, -182.0317) centre (196.0506, -196.3238) ccw
  arc A79 (118.0074, -180.5241) -> (135.3962, -182.0317) centre (130.9156, -132.6777) ccw
  arc A80 (118.0074, -180.5241) -> (89.9158, -208.4836) centre (145.6392, -236.3783) ccw
  arc A81 (73.3667, -203.0191) -> (89.9158, -208.4836) centre (96.9378, -159.4266) ccw
  arc A82 (73.3667, -203.0191) -> (39.5226, -223.7609) centre (87.311, -263.7543) ccw
  arc A83 (24.6991, -214.6443) -> (39.5226, -223.7609) centre (57.6686, -177.6456) ccw
  arc A84 (24.6991, -214.6443) -> (-13.078, -227.0215) centre (24.1992, -276.9578) ccw
  arc A85 (-25.3851, -214.7528) -> (-13.078, -227.0215) centre (15.2139, -186.3341) ccw
  arc A86 (-25.3851, -214.7528) -> (-65.0567, -218.07) centre (-40.3004, -275.2569) ccw
  arc A87 (-74.1937, -203.3165) -> (-65.0567, -218.07) centre (-28.1443, -185.0038) ccw
  arc A88 (-74.1937, -203.3165) -> (-113.6132, -197.3686) centre (-102.7124, -258.7232) ccw
  arc A89 (-119.098, -180.9293) -> (-113.6132, -197.3686) centre (-70.0702, -173.7063) ccw
  arc A90 (-119.098, -180.9293) -> (-156.1268, -166.0136) centre (-159.6693, -228.2283) ccw
  arc A91 (-157.6747, -148.7758) -> (-156.1268, -166.0136) centre (-108.3007, -153.0308) ccw
  arc A92 (-157.6747, -148.7758) -> (-190.2985, -125.6774) centre (-208.0931, -185.3981) ccw
  arc A93 (-187.8364, -108.5689) -> (-190.2985, -125.6774) centre (-140.7674, -124.074) ccw
  arc A94 (-187.8364, -108.5689) -> (-214.275, -78.519) centre (-245.3625, -132.5263) ccw
  arc A95 (-207.9454, -62.4584) -> (-214.275, -78.519) centre (-165.7093, -88.3816) ccw
  arc A96 (-207.9454, -62.4584) -> (-226.75, -27.0687) centre (-269.4545, -72.4509) ccw
  arc A97 (-226.75, 26.7439) -> (-207.9454, 62.1336) centre (-269.4545, 72.1261) ccw
  arc A98 (-214.275, 78.1942) -> (-207.9454, 62.1336) centre (-165.7093, 88.0568) ccw
  arc A99 (-214.275, 78.1942) -> (-187.8364, 108.2441) centre (-245.3625, 132.2015) ccw
  arc A100 (-190.2985, 125.3526) -> (-187.8364, 108.2441) centre (-140.7674, 123.7492) ccw
  arc A101 (-190.2985, 125.3526) -> (-157.6747, 148.451) centre (-208.0931, 185.0733) ccw
  arc A102 (-156.1268, 165.6888) -> (-157.6747, 148.451) centre (-108.3007, 152.706) ccw
  arc A103 (-156.1268, 165.6888) -> (-119.098, 180.6045) centre (-159.6693, 227.9035) ccw
  arc A104 (-113.6132, 197.0438) -> (-119.098, 180.6045) centre (-70.0702, 173.3815) ccw
  arc A105 (-113.6132, 197.0438) -> (-74.1937, 202.9917) centre (-102.7124, 258.3984) ccw
  arc A106 (-226.75, 26.7439) -> (-211.8149, -0.1624) centre (-178.2865, 36.0467) ccw
  arc A107 (-211.8149, -0.1624) -> (-226.75, -27.0687) centre (-174.0425, -38.7272) ccw
  point P0 (0, 0)
  dimension "d16" = 12.7
  constraints: 108 point on circle, 54 centre point, 49 other
  measures "d16" radial gap between concentric circles of A53 A105
extrude "Extrusion4" add sketch "Sketch4" along normal blind 6.35 contours A55 A56 A57 A58 A59 A60 A61 A62 A63 A64 A65 A66 A67 A68 A69 A70 A71 A72 A73 A74 A75 A76 A77 A78 A79 A80 A81 A82 A83 A84 A85 A86 A87 A88 A89 A90 A91 A92 A93 A94 A95 A96 A107 A106 A97 A98 A99 A100 A101 A102 A103 A104 A105 A54
sketch "Sketch5" plane through (0, 25.4, 0) normal (0, 1, 0) x (1, 0, 0)
  arc A0 (-0.8471, -12.7) -> (-60.7152, -36.6072) centre (-0.8471, -99.6142) ccw
  arc A1 (57.292, -58.8333) -> (-0.8471, -12.7) centre (-21.0595, -97.8739) ccw
  arc A2 (-34.7456, -103.9573) -> (22.4011, -110.3267) centre (18.0973, 110.6042) ccw
  arc A3 (-60.7152, -36.6072) -> (-34.7456, -103.9573) centre (-24.4681, -61.3125) ccw
  arc A4 (22.4011, -110.3267) -> (57.292, -58.8333) centre (14.2515, -67.2373) ccw
  line L0 (375.0548, 0) -> (-376.8381, 0) projected
  arc A5 (-60.7152, 36.6072) -> (-0.8471, 12.7) centre (-0.8471, 99.6142) ccw
  arc A6 (-0.8471, 12.7) -> (57.292, 58.8333) centre (-21.0595, 97.8739) ccw
  arc A7 (22.4011, 110.3267) -> (-34.7456, 103.9573) centre (18.0973, -110.6042) ccw
  arc A8 (-34.7456, 103.9573) -> (-60.7152, 36.6072) centre (-24.4681, 61.3125) ccw
  arc A9 (57.292, 58.8333) -> (22.4011, 110.3267) centre (14.2515, 67.2373) ccw
  dimension "d30" = 43.8658
  dimension "d36" = 87.5393
  dimension "d37" = 220.9729
  dimension "d38" = 43.8533
  dimension "d60" = 12.7
  constraints: 20 point on circle, 10 centre point, 10 symmetric about line, 5 other
  measures "d30" radius of A3
  measures "d36" radius of A1
  measures "d37" radius of A2
  measures "d38" radius of A4
  measures "d60" distance from line of L0 A0.start
extrude "Extrusion5" add sketch "Sketch5" along normal blind 6.35
ref_plane "Work Plane1" through (-12.7, 38.1, 46.0375) normal (0, 1, 0) x (1, 0, 0)
sketch "Sketch8" plane through (0, 31.75, 0) normal (0, 1, 0) x (1, 0, 0)
  circle A0 centre (-12.7, 46.0375) radius 15.875
  circle A1 centre (-12.7, -46.0375) radius 15.875
  point P0 (0, 0)
  constraints: 2 centre point
extrude "Extrusion7" cut sketch "Sketch8" against normal blind 6.35
body "Solid1"
